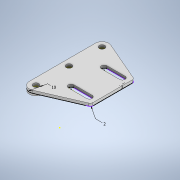
# Autodesk Inventor part: straigthener fixture
Saved by Autodesk Inventor 2022.2 (Build 262287000, 287)
## iProperties
Created: 2022-08-09
Part Number: straigthener fixture
Material: Generic
Document SubType Name: Modeling
Designer: Ilewicz
Density: 1 g/cm^3
Appearance: Default
Author: Ilewicz
Autodesk Inventor part; units mm, degrees
ref_plane "YZ Plane" through (0, 0, 0) normal (1, 0, 0) x (0, 1, 0)
ref_plane "XZ Plane" through (0, 0, 0) normal (0, 1, 0) x (-1, 0, 0)
ref_plane "XY Plane" through (0, 0, 0) normal (0, 0, 1) x (1, 0, 0)
derived "Straigthener.ipt"
sketch "Sketch1" plane through (0, 0, 0) normal (0, 1, 0) x (-1, 0, 0)
  line L0 (41, 0) -> (41, -73)
  line L1 (41, -73) -> (0, -73)
  line L2 (0, -73) -> (0, 0)
  circle A0 centre (35, -67) radius 10 construction
  circle A1 centre (35, -67) radius 3.96
  circle A2 centre (35, -67) radius 2.1
  circle A3 centre (35, -42) radius 10 construction
  circle A4 centre (35, -42) radius 3.96
  circle A5 centre (35, -42) radius 2.1
  circle A6 centre (35, -17) radius 10 construction
  circle A7 centre (35, -17) radius 3.96
  circle A8 centre (35, -17) radius 2.1
  circle A9 centre (14, -54.5) radius 10 construction
  circle A10 centre (14, -54.5) radius 3.96
  circle A11 centre (14, -54.5) radius 2.1
  line L3 (24, -139.1024) -> (24, 22.6885) construction
  line L4 (25, -134.9846) -> (25, 23.5885) construction
  line L5 (14, -54.5) -> (40.7035, -54.5) construction
  line L6 (45.7035, -42) -> (0, -42) construction
  line L7 (19, -49.5) -> (19, -59.5)
  line L8 (19, -59.5) -> (23, -59.5)
  line L9 (23, -59.5) -> (23, -49.5)
  line L10 (23, -49.5) -> (19, -49.5)
  line L11 (9, -59.5) -> (5, -59.5)
  line L12 (5, -59.5) -> (5, -49.5)
  line L13 (5, -49.5) -> (9, -49.5)
  line L14 (9, -49.5) -> (9, -59.5)
  line L15 (14, -122.6698) -> (14, 13.6698)
  line L16 (23, -34.5) -> (19, -34.5)
  line L17 (14, -29.5) -> (40.7035, -29.5) construction
  circle A12 centre (14, -29.5) radius 2.1
  line L18 (23, -24.5) -> (23, -34.5)
  line L19 (19, -34.5) -> (19, -24.5)
  line L20 (14, 38.6698) -> (14, -97.6698)
  circle A13 centre (14, -29.5) radius 3.96
  circle A14 centre (14, -29.5) radius 10 construction
  line L21 (9, -34.5) -> (9, -24.5)
  line L22 (5, -34.5) -> (9, -34.5)
  line L23 (5, -24.5) -> (5, -34.5)
  line L24 (9, -24.5) -> (5, -24.5)
  line L25 (0, -11) -> (0, -84)
  line L26 (19, -24.5) -> (23, -24.5)
  circle A15 centre (35, -67) radius 5
  circle A16 centre (14, -54.5) radius 5
  circle A17 centre (35, -42) radius 5
  circle A18 centre (35, -17) radius 5
  circle A19 centre (14, -29.5) radius 5
  line L27 (19, -24.5) -> (9, -24.5)
  line L28 (19, -34.5) -> (9, -34.5)
  line L29 (41, -7) -> (0, -7)
  line L30 (41, 0) -> (0, 0)
  circle A20 centre (30, -3.5) radius 2
  circle A21 centre (11, -3.5) radius 2
  line L31 (47, -3.5) -> (-4, -3.5)
sketch "Sketch2" plane through (0, 0, 0) normal (0, 1, 0) x (-1, 0, 0)
  circle A0 centre (35, -17) radius 2.1 projected
  circle A1 centre (35, -17) radius 3.96 construction
  circle A2 centre (35, -42) radius 2.1 projected
  circle A3 centre (35, -42) radius 3.96 construction
  circle A4 centre (35, -67) radius 2.1 projected
  circle A5 centre (35, -67) radius 3.96 construction
  line L0 (14, -29.5) -> (40.7035, -29.5) construction
  line L1 (14, -54.5) -> (40.7035, -54.5) construction
  line L2 (23, -24.5) -> (23, -34.5) projected
  line L3 (5, -24.5) -> (5, -34.5) projected
  line L4 (5, -59.5) -> (5, -49.5) projected
  line L5 (23, -59.5) -> (23, -49.5) projected
  circle A6 centre (35, -17) radius 5
  circle A7 centre (35, -42) radius 5
  circle A8 centre (35, -67) radius 5
  arc A9 (20.9, -31.6) -> (20.9, -27.4) centre (20.9, -29.5) ccw
  arc A10 (7.1, -27.4) -> (7.1, -31.6) centre (7.1, -29.5) ccw
  arc A11 (7.1, -52.4) -> (7.1, -56.6) centre (7.1, -54.5) ccw
  arc A12 (20.9, -56.6) -> (20.9, -52.4) centre (20.9, -54.5) ccw
  line L6 (20.9, -27.4) -> (7.1, -27.4)
  line L7 (7.1, -31.6) -> (20.9, -31.6)
  line L8 (20.9, -52.4) -> (7.1, -52.4)
  line L9 (7.1, -56.6) -> (20.9, -56.6)
  line L10 (5, -24.5) -> (33.019, -12.4092)
  line L11 (5, -59.5) -> (33.019, -71.5908)
  line L12 (39.9991, -67.0954) -> (39.9991, -17.0954)
  line L13 (2, -27.1098) -> (2, -56.8902)
  line L14 (3.2076, -58.7265) -> (5, -59.5)
  line L15 (3.2076, -25.2735) -> (5, -24.5)
  arc A13 (3.2076, -25.2735) -> (2, -27.1098) centre (4, -27.1098) ccw
  arc A14 (2, -56.8902) -> (3.2076, -58.7265) centre (4, -56.8902) ccw
  point P0 (0, 0)
  point P1 (5, -29.5)
  point P2 (5, -54.5)
  point P3 (39.9991, -66.9046)
  point P4 (39.9991, -42.0954)
  point P5 (39.9991, -41.9046)
  point P6 (5, -54.5)
  dimension "d1" = 10
  dimension "d6" = 2
  dimension "d7" = 3
  constraints: 20 end point, 16 point on circle, 10 tangent, 9 centre point, 7 equal radius, 4 point on line, 3 coincident, 3 parallel, 1 horizontal, 1 midpoint, 1 vertical
  measures "d1" diameter of A6
  measures "d6" radius of A13
  measures "d7" distance from line of L13 point (5, -54.5)
extrude "Extrusion1" add sketch "Sketch2" along normal blind 2 contours A6 | A7 | A6 L12 A8 L11 L14 A14 L13 A13 L15 L10 | A8
extrude "Extrusion2" add sketch "Sketch2" against normal blind 1.5 contours A6 | A7 | A8
body "Solid1"
